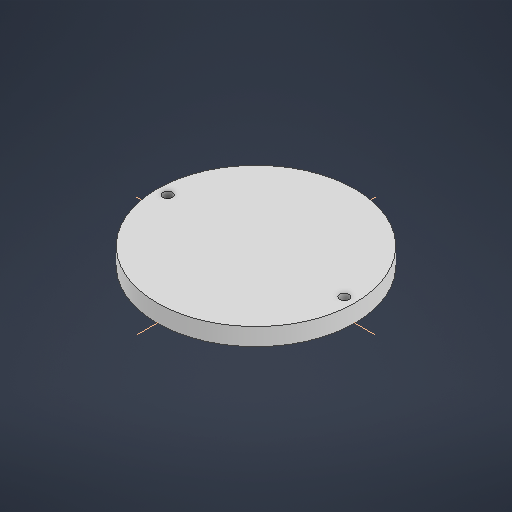
# Autodesk Inventor part: Build Plate with 35mm FOV Sketch
Saved by Autodesk Inventor 2026.2 (Build 302298000, 298)
## iProperties
Created: 2026-03-26
Part Number: Build Plate with 35mm FOV Sketch
Material: Generic
Document SubType Name: Modeling
Designer: mumin
Density: 1 g/cm^3
Appearance: Default
Author: mumin
Autodesk Inventor part; units mm, degrees
ref_plane "YZ Plane" through (0, 0, 0) normal (1, 0, 0) x (0, 1, 0)
ref_plane "XZ Plane" through (0, 0, 0) normal (0, 1, 0) x (-1, 0, 0)
ref_plane "XY Plane" through (0, 0, 0) normal (0, 0, 1) x (1, 0, 0)
sketch "Sketch1" plane through (0, 0, 0) normal (0, 1, 0) x (-1, 0, 0)
  circle A0 centre (0, 0) radius 85
  dimension "d0" = 170
  constraints: 1 centre point, 1 coincident
  measures "d0" diameter of A0
extrude "Extrusion1" add sketch "Sketch1" along normal blind 15
sketch "Sketch2" plane through (0, 15, 0) normal (0, 1, 0) x (1, 0, 0)
  circle A0 centre (0, 0) radius 85 projected
  line L0 (51, -22.7944) -> (-51, -22.7944)
  line L1 (-56, 50.2056) -> (56, 50.2056)
  line L2 (0, 119) -> (0, -119) projected
  line L3 (-56, 50.2056) -> (51, -22.7944) construction
  line L4 (56, 50.2056) -> (-51, -22.7944) construction
  line L5 (-56, 50.2056) -> (-51, -22.7944)
  line L6 (56, 50.2056) -> (51, -22.7944)
  line L7 (-119, 0) -> (119, 0) projected
  point P0 (0, -22.7944)
  point P1 (0, 50.2056)
  point P2 (0, 12)
  dimension "d4" = 112
  dimension "d5" = 73
  dimension "d7" = 102
  dimension "d9" = 12
  constraints: 12 end point, 4 point on line, 2 midpoint, 1 horizontal, 1 parallel
  measures "d4" distance of L1.start L1.end
  measures "d5" distance between parallel lines of L0 L1
  measures "d7" distance of L0.start L0.end
  measures "d9" distance from line of L7 point (0, 12)
sketch "Sketch3" plane through (0, 15, 0) normal (0, 1, 0) x (1, 0, 0)
  circle A0 centre (0, 0) radius 76
  point P0 (-76, 0)
  point P1 (76, 0)
  dimension "d10" = 152
  constraints: 2 point on circle, 1 centre point, 1 coincident
  measures "d10" diameter of A0
hole "Hole1" at (-76, 15, 0) at (76, 15, 0) direction (0, -1, 0) diameter 4.5 depth 15 counterbore diameter 8 counterbore depth 12
body "Solid1"
